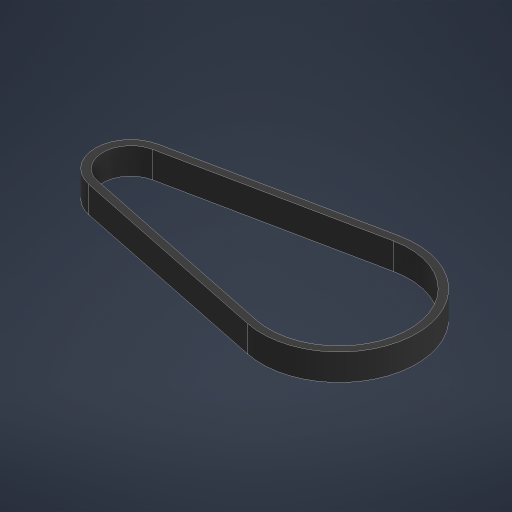
# Autodesk Inventor part: CLIM_004_RollerBelt
Saved by Autodesk Inventor 2024.2 (Build 282272000, 272)
## iProperties
Created: 2024-08-08
Part Number: CLIM_004_RollerBelt
Material: Rubber, Silicone
Document SubType Name: Modeling
Designer: Bryan
Density: 1.25 g/cm^3
Appearance: Rubber - Black
Author: Bryan
Autodesk Inventor part; units mm, degrees
ref_plane "YZ Plane" through (0, 0, 0) normal (1, 0, 0) x (0, 1, 0)
ref_plane "XZ Plane" through (0, 0, 0) normal (0, 1, 0) x (-1, 0, 0)
ref_plane "XY Plane" through (0, 0, 0) normal (0, 0, 1) x (1, 0, 0)
sketch "Sketch1" plane through (0, 0, 0) normal (0, 1, 0) x (-1, 0, 0)
  circle A0 centre (0, 0) radius 23.876 construction
  circle A1 centre (71.0438, 0) radius 9.5504 construction
  line L0 (72.9696, 9.3542) -> (4.8145, 23.3856)
  line L1 (72.9696, -9.3542) -> (4.8145, -23.3856)
  arc A2 (72.9696, -9.3542) -> (72.9696, 9.3542) centre (71.0438, 0) ccw
  arc A3 (4.8145, 23.3856) -> (4.8145, -23.3856) centre (0, 0) ccw
  line L2 (5.3266, 25.8734) -> (73.4818, 11.842)
  arc A4 (73.4818, -11.842) -> (73.4818, 11.842) centre (71.0438, 0) ccw
  line L3 (73.4818, -11.842) -> (5.3266, -25.8734)
  arc A5 (5.3266, 25.8734) -> (5.3266, -25.8734) centre (0, 0) ccw
  dimension "d0" = 47.752
  dimension "d1" = 19.1008
  dimension "d2" = 71.0438
  dimension "d3" = 2.54
  constraints: 12 point on circle, 8 end point, 8 tangent, 6 centre point, 1 coincident, 1 horizontal alignment, 3 other
  measures "d0" diameter of A0
  measures "d1" diameter of A1
  measures "d2" distance of point (0, 0) A1.centre
  measures "d3" distance between parallel lines of L0 L2
extrude "Extrusion1" add sketch "Sketch1" along normal blind 9
body "Solid1"
